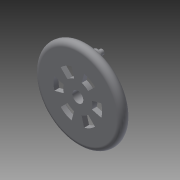
# Autodesk Inventor part: Wheel
Saved by Autodesk Inventor 2015 (Build 190159000, 159)
## iProperties
Created: 2018-03-27
Part Number: Wheel
Material: Generic
Document SubType Name: Modeling
Designer: Administrator
Density: 1 g/cm^3
Appearance: Default
Mass: 11.5439 g
Surface Area: 63.3048 cm^2
Volume: 11.5439 cm^3
Author: Administrator
Autodesk Inventor part; units mm, degrees
ref_plane "YZ Plane" through (0, 0, 0) normal (1, 0, 0) x (0, 1, 0)
ref_plane "XZ Plane" through (0, 0, 0) normal (0, 1, 0) x (-1, 0, 0)
ref_plane "XY Plane" through (0, 0, 0) normal (0, 0, 1) x (1, 0, 0)
sketch "Sketch1" plane through (0, 0, 0) normal (0, 1, 0) x (-1, 0, 0)
  line L0 (-3.556, 0) -> (-25.4, 0)
  line L1 (-3.556, 0) -> (-3.556, -6.35)
  arc A0 (-25.4, 0) -> (-25.4, -6.35) centre (-25.4, -3.175) ccw
  line L2 (-25.4, -6.35) -> (-19.05, -6.35)
  line L3 (-19.05, -3.175) -> (-6.35, -3.175)
  line L4 (0, 0) -> (0, -1.459) construction
  line L5 (-19.05, -6.35) -> (-19.05, -3.175)
  line L6 (-3.556, -6.35) -> (-6.35, -6.35)
  line L7 (-6.35, -6.35) -> (-6.35, -3.175)
  dimension "d0" = 25.4
  dimension "d1" = 3.556
  dimension "d2" = 6.35
  dimension "d3" = 0
  dimension "d5" = 3.175
  dimension "d6" = 6.35
  dimension "d9" = 12.7
  dimension "d11" = 3.175
  constraints: 16 end point, 4 horizontal, 2 perpendicular, 2 point on circle, 2 tangent, 2 vertical, 1 centre point
  measures "d0" distance of L0.end L4.start
  measures "d1" distance from line of L4.start L1
  measures "d2" distance of L0.start L1.end
  measures "d3" distance from line of L4.start L0
  measures "d5" radius of A0
  measures "d6" distance of L2.start L2.end
  measures "d9" distance of L3.start L3.end
  measures "d11" distance between parallel lines of L0 L3
revolve "Revolution1" add sketch "Sketch1" angle 360 about axis through (0, 0, 0) along (0, 0, -1)
fillet "Fillet1" radius 1.5875 4 edges at (-6.35, 0, -3.175) (-6.35, 0, -6.35) (-19.05, 0, -6.35) (-19.05, 0, -3.175)
sketch "Sketch2" plane through (0, 0, 0) normal (0, 0, 1) x (1, 0, 0)
  circle A0 centre (0, 0) radius 25.4 projected
  circle A1 centre (0, 0) radius 3.556 projected
  arc A2 (-9.2004, 2.4653) -> (-9.2004, -2.4653) centre (0, 0) ccw
  arc A3 (-15.3341, 4.1088) -> (-15.3341, -4.1088) centre (0, 0) ccw
  line L0 (0, 0) -> (0, 7.9375) construction
  line L1 (-9.2004, -2.4653) -> (-15.3341, -4.1088)
  line L2 (-9.2004, 2.4653) -> (-15.3341, 4.1088)
  arc A4 (-6.7352, -6.7352) -> (-2.4653, -9.2004) centre (0, 0) ccw
  arc A5 (-11.2253, -11.2253) -> (-4.1088, -15.3341) centre (0, 0) ccw
  line L3 (-2.4653, -9.2004) -> (-4.1088, -15.3341)
  line L4 (-6.7352, -6.7352) -> (-11.2253, -11.2253)
  arc A6 (2.4653, -9.2004) -> (6.7352, -6.7352) centre (0, 0) ccw
  arc A7 (4.1088, -15.3341) -> (11.2253, -11.2253) centre (0, 0) ccw
  line L5 (6.7352, -6.7352) -> (11.2253, -11.2253)
  line L6 (2.4653, -9.2004) -> (4.1088, -15.3341)
  arc A8 (9.2004, -2.4653) -> (9.2004, 2.4653) centre (0, 0) ccw
  arc A9 (15.3341, -4.1088) -> (15.3341, 4.1088) centre (0, 0) ccw
  line L7 (9.2004, 2.4653) -> (15.3341, 4.1088)
  line L8 (9.2004, -2.4653) -> (15.3341, -4.1088)
  arc A10 (6.7352, 6.7352) -> (2.4653, 9.2004) centre (0, 0) ccw
  arc A11 (11.2253, 11.2253) -> (4.1088, 15.3341) centre (0, 0) ccw
  line L9 (2.4653, 9.2004) -> (4.1088, 15.3341)
  line L10 (6.7352, 6.7352) -> (11.2253, 11.2253)
  arc A12 (-2.4653, 9.2004) -> (-6.7352, 6.7352) centre (0, 0) ccw
  arc A13 (-4.1088, 15.3341) -> (-11.2253, 11.2253) centre (0, 0) ccw
  line L11 (-6.7352, 6.7352) -> (-11.2253, 11.2253)
  line L12 (-2.4653, 9.2004) -> (-4.1088, 15.3341)
  dimension "d14" = 19.05
  dimension "d15" = 31.75
  dimension "d18" = 75
  dimension "d19" = 105
  dimension "d22" = 360
  constraints: 26 end point, 24 point on circle, 12 centre point, 7 coincident, 1 vertical, 61 other
  measures "d14" diameter of A2
  measures "d15" diameter of A3
  measures "d18" angle of L0 L2
  measures "d19" angle of L0 L1
extrude "Extrusion1" cut sketch "Sketch2" against normal blind 25.4 contours A2 L1 A3 L2 | A4 L3 A5 L4 | A6 L5 A7 L6 | A8 L7 A9 L8 | A10 L9 A11 L10 | A12 L11 A13 L12
sketch "Sketch3" plane through (0, 0, -3.175) normal (0, 0, -1) x (-1, 0, 0)
  circle A0 centre (0, 17.78) radius 3.175
  circle A1 centre (0, 17.78) radius 1.5875
  point P0 (0, 0)
  dimension "d26" = 17.78
  dimension "d27" = 6.35
  dimension "d28" = 17.78
  dimension "d29" = 3.175
  constraints: 2 centre point
  measures "d26" distance of point (0, 0) A0.centre
  measures "d27" diameter of A0
  measures "d28" distance of point (0, 0) A1.centre
  measures "d29" diameter of A1
extrude "Extrusion2" add sketch "Sketch3" along normal blind 9.525
extrude "Extrusion3" add sketch "Sketch3" along normal blind 12.7 contours A1
sketch "Sketch4" plane through (0, 17.78, -15.875) normal (0, 0, -1) x (-1, 0, 0)
  point P0 (0, -17.78)
  point P1 (0, 0)
hole "Hole1" at (0, 17.78, -15.875) direction (0, 0, 1) diameter 1.5875 depth 6.35 tip angle 118
body "Solid1"
